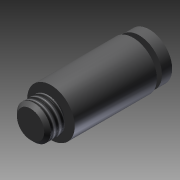
# Autodesk Inventor part: KQ2S23-M5N N
Saved by Autodesk Inventor 2016 (Build 200138000, 138)
## iProperties
Category: PARTsolutions
Company: SMC
Created: 2015-04-13
Part Number: KQ2S23-M5N N
Catalog Web Link: www.cadenas.de
Description: KQ2S-Hex. Socket Head Male Connector (Gasket Seal)
Vendor: SMC
Document SubType Name: Modeling
Designer: PARTuser1
Manufacturer: SMC
Mass: 2.6 g
Surface Area: 6.37668 cm^2
Volume: 0.467592 cm^3
Density: 1 g/cm^3
Material: Generic
Appearance: PSOLRGB-175-175-175
PSOL_IDENT_0: {$CADENAS_DATA\23d-libs\smc_jp\fittings_and_tubing\fittings_for_general_purposes\kq2_new\kq2_1\kq2s_
PSOL_IDENT_1: hshmc_gs.prj},168 {VTYP=3D},{NB=KQ2S23-M5N},{LINA=KQ2S23-M5N},{NN=KQ2S},{DATE=17.03.2015 08:12:56},{
PSOL_IDENT_2: GEOMDATE=30.06.2014 06:14:02},{VERSION=},{LINEID=30},{LINESUBID=-1},{WBVAR=MATERIAL}  {NB=KQ2S23-M5N
PSOL_IDENT_3: },{LINA=KQ2S23-M5N},{KT=DUMMY},{GUI=KQ2S23-M5},{OD=3.2},{T=M5x0.8},{RA=5},{RP=0.8},{RL=3},{MODEL=KQ2
PSOL_IDENT_4: S23-M5N},{MATERIAL=N},{MATERIALX='A','(A) Brass','N','(N) Brass + With electroless nickel plating'},
PSOL_IDENT_5: {TUBE=23},{PORT=M5},{H=2.0},{D=7.0},{L1=17.5},{L2=16.3},{A=14.5},{M=13.3},{EA1=2.5},{EA2=2.5},{MBS=2
PSOL_IDENT_6: .0},{CNSMASSEXACT=2.6},{NENN=KQ2S23-M5N},{A1=6.7},{A2=3.95}
SUPPLIER: SMC
ARTICLENO: KQ2S23-M5N
BOMINFO: KQ2S23-M5N
CREATOR: CADENAS GmbH
Title: KQ2S23-M5N
Author: Cadenas PARTsolutions
Comments: Hex. Socket Head Male Connector (Gasket Seal)
Autodesk Inventor part; units mm, degrees
ref_plane "YZ Plane" through (0, 0, 0) normal (1, 0, 0) x (0, 1, 0)
ref_plane "XZ Plane" through (0, 0, 0) normal (0, 1, 0) x (-1, 0, 0)
ref_plane "XY Plane" through (0, 0, 0) normal (0, 0, 1) x (1, 0, 0)
sketch "Sketch_1" plane through (0, 0, 0) normal (0, 0, 1) x (1, 0, 0)
  line L0 (0, -3) -> (0, 14.5)
  line L1 (0, 14.5) -> (3.35, 14.5)
  line L2 (3.35, 14.5) -> (3.35, 13)
  line L3 (3.35, 13) -> (1.975, 13)
  line L4 (1.975, 13) -> (1.975, 12.1)
  line L5 (1.975, 12.1) -> (3.5, 12.1)
  line L6 (3.5, 12.1) -> (3.5, 0)
  line L7 (3.5, 0) -> (2.0095, 0)
  line L8 (2.0095, 0) -> (2.5, -0.4905)
  line L9 (2.5, -0.4905) -> (2.5, -2.5095)
  line L10 (2.5, -2.5095) -> (2.0095, -3)
  line L11 (2.0095, -3) -> (0, -3)
  line L12 (0, -3) -> (0, 14.5)
  constraints: 26 end point
revolve "Revolution1" add sketch "Sketch_1" angle 360 about axis through (0, -3, 0) along (0, -1, 0)
thread "Thread1" size "M5x0.8" class "6g" standard "ISO Metric profile" full length
sketch "Sketch_2" plane through (0, 0, 0) normal (0, 0, 1) x (1, 0, 0)
  line L0 (0, 1.2) -> (0, 14.5)
  line L1 (0, 14.5) -> (1.6, 14.5)
  line L2 (1.6, 14.5) -> (1.6, 1.2)
  line L3 (1.6, 1.2) -> (0, 1.2)
  line L4 (0, 1.2) -> (0, 14.5)
  constraints: 10 end point
revolve "Revolution2" cut sketch "Sketch_2" angle 360 about axis through (0, 1.2, 0) along (0, -1, 0)
sketch "Sketch_3" plane through (0, 14.5, 0) normal (0, 1, 0) x (1, 0, 0)
  line L0 (-1, 0.5774) -> (-1, -0.5774)
  line L1 (-1, -0.5774) -> (0, -1.1547)
  line L2 (0, -1.1547) -> (1, -0.5774)
  line L3 (1, -0.5774) -> (1, 0.5774)
  line L4 (1, 0.5774) -> (0, 1.1547)
  line L5 (0, 1.1547) -> (-1, 0.5774)
  constraints: 12 end point
extrude "Extrusion1" cut sketch "Sketch_3" against normal blind 16.3
body "Solid1"
